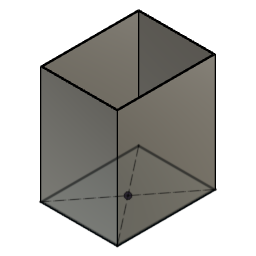
Dust caps Optic array v2 (Autodesk Fusion 360 design; units mm, degrees)
Autodesk Fusion 360 part; units mm, degrees
sketch "Sketch1" plane through (0, 0, 0) normal (0, 0, 1) x (1, 0, 0)
  line L0 (35, 45) -> (-35, 45)
  line L1 (-35, 45) -> (-35, -45)
  line L2 (-35, -45) -> (35, -45)
  line L3 (35, -45) -> (35, 45)
  line L4 (35, 45) -> (-35, -45) construction
  line L5 (-35, 45) -> (35, -45) construction
  line L6 (36, 46) -> (-36, 46)
  line L7 (-36, 46) -> (-36, -46)
  line L8 (-36, -46) -> (36, -46)
  line L9 (36, -46) -> (36, 46)
  line L10 (36, 46) -> (-36, -46) construction
  line L11 (-36, 46) -> (36, -46) construction
  dimension "d1" = 70
  dimension "d2" = 90
  dimension "d3" = 72
  dimension "d4" = 92
  constraint horizontal L0
  constraint perpendicular L0 L1
  constraint parallel L0 L2
  constraint parallel L1 L3
  constraint coincident L4 origin
  constraint coincident L5 origin
  constraint horizontal L6
  constraint perpendicular L6 L7
  constraint parallel L6 L8
  constraint parallel L7 L9
  constraint coincident L10 origin
  constraint coincident L11 origin
  measures "d1" distance of L1.end L2.end
  measures "d2" distance of L0.end L1.end
  measures "d3" distance of L7.end L8.end
  measures "d4" distance of L6.end L7.end
extrude "Extrude1" add sketch "Sketch1" along normal blind 1 contours L0 L1 L2 L3
extrude "Extrude2" add sketch "Sketch1" along normal blind 110
